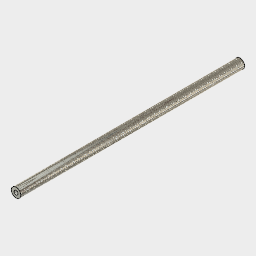
Bed_Base_v2 (Autodesk Fusion 360 archive; units mm, degrees)
design "Y Axis Shaft"
Autodesk Fusion 360 part; units mm, degrees
note: some values were not read from the file. Chosen so that the rebuilt part matches the saved one: how an offset face is resized.
sketch "Sketch1" plane through (0, 0, 0) normal (0, 1, 0) x (1, 0, 0) in component "Y Axis Shaft"
  circle A0 centre (0, 0) radius 4
  circle A1 centre (0, 0) radius 2
  dimension "d1" = 8
  dimension "d2" = 4
  measures "d1" diameter of A0
  measures "d2" diameter of A1
extrude "Extrude1" add sketch "Sketch1" along normal mid plane 187 contours A0 | A1 in component "Y Axis Shaft"
extrude "Extrude2" cut sketch "Sketch1" along normal blind 9 from surface at -93.5 contours A1 in component "Y Axis Shaft"
extrude "Extrude3" cut sketch "Sketch1" against normal blind 9 from surface at 93.5 contours A1 in component "Y Axis Shaft"
thread "Thread1" "ISO Metric profile 4.0 M4x0.7 6H" major diameter 4.1095 minor diameter 3.332 pitch 0.7 angle 60 resizes the face on face at (1.9975, 87.5, 0.0997) in component "Y Axis Shaft"
thread "Thread2" "ISO Metric profile 4.0 M4x0.7 6H" major diameter 4.1095 minor diameter 3.332 pitch 0.7 angle 60 resizes the face on face at (1.9975, -90.5, -0.0997) in component "Y Axis Shaft"
component "Y Axis Shaft" placed x (1, 0, 0) y (0, 1, 0) z (0, 0, 1) at (0, 0, 0)
equation "d3 = ( 187 / 2 ) * 1 mm"

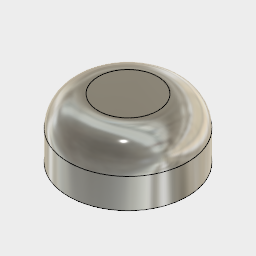
design "Bed Rod Screw Caps"
Autodesk Fusion 360 part; units mm, degrees
sketch "Sketch1" plane through (0, 0, 0) normal (0, 0, 1) x (1, 0, 0) in component "Bed Rod Screw Caps"
  circle A0 centre (0, 0) radius 4
  dimension "d1" = 8
  measures "d1" diameter of A0
extrude "Extrude1" add sketch "Sketch1" along normal blind 4 in component "Bed Rod Screw Caps"
fillet "Fillet1" radius 2 1 edges at (-3.7293, -1.4465, 4) in component "Bed Rod Screw Caps"
component "Bed Rod Screw Caps" placed x (1, 0, 0) y (0, 1, 0) z (0, 0, 1) at (0, 0, 0)

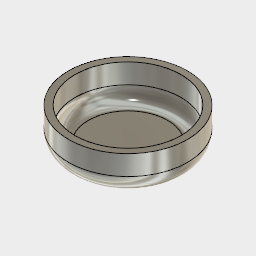
design "Bed Spring Cap"
Autodesk Fusion 360 part; units mm, degrees
sketch "Sketch1" plane through (0, 0, 0) normal (0, 1, 0) x (1, 0, 0) in component "Bed Spring Cap"
  arc A0 (4.5, -1.5) -> (3, 0) centre (3, -1.5) ccw
  arc A1 (-3, 0) -> (-4.5, -1.5) centre (-3, -1.5) ccw
  arc A2 (4, -1.5) -> (3, -0.5) centre (3, -1.5) ccw
  arc A3 (-3, -0.5) -> (-4, -1.5) centre (-3, -1.5) ccw
  line L0 (4.5, -1.5) -> (4.5, -3)
  line L1 (0, 0) -> (0, -0.5)
  line L2 (4, -3) -> (4.5, -3)
  line L3 (4, -1.5) -> (4, -3)
  line L4 (-3, -0.5) -> (3, -0.5)
  line L5 (-4, -3) -> (-4, -1.5)
  line L6 (-3, 0) -> (3, 0)
  line L7 (-4.5, -3) -> (-4, -3)
  line L8 (-4.5, -3) -> (-4.5, -1.5)
  dimension "d7" = 1.5
  dimension "d8" = 6
  dimension "d9" = 3
  dimension "d10" = 1
  dimension "d11" = 1.5
  measures "d7" radius of A0
  measures "d8" distance of A1.start A0.end
  measures "d9" distance of L7.start L6
  measures "d10" radius of A2
  measures "d11" distance of L7.start A1.end
revolve "Revolve1" add sketch "Sketch1" angle 360 about axis through (0, 0, 0) along (0, 0, 1) contours A1 A3 L1 L4 L5 L6 L7 L8 in component "Bed Spring Cap"
component "Bed Spring Cap" placed x (1, 0, 0) y (0, 1, 0) z (0, 0, 1) at (0, 0, 0)
